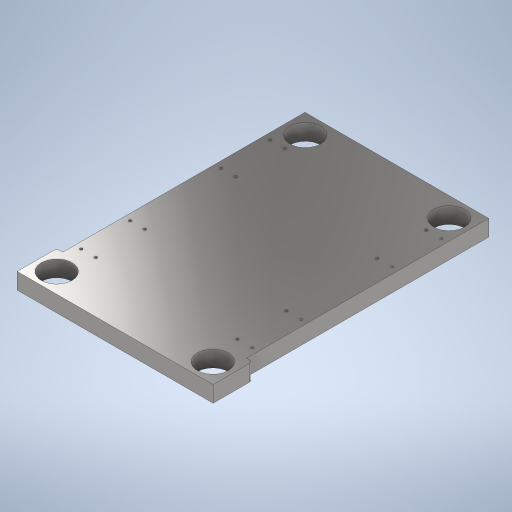
# Autodesk Inventor part: Weight Frame Top
Saved by Autodesk Inventor 2023 (Build 270158000, 158)
## iProperties
Created: 2022-10-18
Part Number: Weight Frame Top
Material: Stainless Steel
Document SubType Name: Modeling
Designer: Hayden Swanson
Density: 8 g/cm^3
Appearance: Semi-Polished
Author: Hayden Swanson
Autodesk Inventor part; units mm, degrees
ref_plane "YZ Plane" through (0, 0, 0) normal (1, 0, 0) x (0, 1, 0)
ref_plane "XZ Plane" through (0, 0, 0) normal (0, 1, 0) x (-1, 0, 0)
ref_plane "XY Plane" through (0, 0, 0) normal (0, 0, 1) x (1, 0, 0)
sketch "Sketch1" plane through (0, 0, 0) normal (0, 1, 0) x (-1, 0, 0)
  line L0 (0, 0) -> (190.5, 0)
  line L1 (190.5, 0) -> (190.5, -292.1)
  line L2 (190.5, -292.1) -> (0, -292.1)
  line L3 (0, -292.1) -> (0, 0)
  line L4 (0, -292.1) -> (-6.35, -292.1)
  line L5 (-6.35, -292.1) -> (-6.35, 0)
  line L6 (-6.35, 0) -> (0, 0)
  line L7 (190.5, -292.1) -> (196.85, -292.1)
  line L8 (196.85, -292.1) -> (196.85, 0)
  line L9 (196.85, 0) -> (190.5, 0)
  dimension "d0" = 190.5
  dimension "d1" = 292.1
  dimension "d259" = 6.35
  dimension "d260" = 6.35
  constraints: 20 end point, 4 perpendicular, 3 horizontal, 3 parallel
  measures "d0" distance of L1.end L2.end
  measures "d1" distance of L0.end L1.end
  measures "d259" distance of L2.end L4.end
  measures "d260" distance of L1.end L7.end
extrude "Extrusion1" add sketch "Sketch1" along normal blind 16.764
sketch "Sketch2" plane through (0, 16.764, 0) normal (0, 1, 0) x (1, 0, 0)
  line L0 (-176.2125, 0) -> (-176.2125, 20.32)
  line L1 (0, 0) -> (-14.2875, 0)
  line L2 (-14.2875, 0) -> (-14.2875, 20.32)
  line L3 (-190.5, 292.1) -> (-169.8625, 292.1)
  line L4 (-169.8625, 292.1) -> (-169.8625, 271.78)
  line L5 (-190.5, 271.78) -> (-190.5, 292.1)
  line L6 (0, 292.1) -> (-20.6375, 292.1)
  line L7 (-20.6375, 292.1) -> (-20.6375, 271.78)
  line L8 (0, 271.78) -> (0, 292.1)
  circle A0 centre (-176.2125, 20.32) radius 15.9766
  circle A1 centre (-14.2875, 20.32) radius 15.9766
  circle A2 centre (-20.6375, 271.78) radius 15.9766
  circle A3 centre (-169.8625, 271.78) radius 15.9766
  line L9 (6.35, 0) -> (6.35, 292.1) projected
  line L10 (6.35, 20.32) -> (-14.2875, 20.32)
  line L11 (-196.85, 292.1) -> (-196.85, 0) projected
  line L12 (-196.85, 20.32) -> (-176.2125, 20.32)
  dimension "d5" = 20.32
  dimension "d7" = 20.32
  dimension "d9" = 20.32
  dimension "d11" = 20.32
  dimension "d12" = 31.9532
  dimension "d14" = 31.9532
  dimension "d15" = 31.9532
  dimension "d264" = 31.9532
  dimension "d274" = 20.6375
  dimension "d276" = 20.6375
  constraints: 22 end point, 4 centre point, 4 coincident, 4 horizontal, 4 perpendicular, 2 parallel, 2 point on line
  measures "d5" distance of L0.end L0.start
  measures "d7" distance of L1.end L2.end
  measures "d9" distance of L3.end L4.end
  measures "d11" distance of L7.end L6.end
  measures "d12" diameter of A0
  measures "d14" diameter of A2
  measures "d15" diameter of A3
  measures "d264" diameter of A1
  measures "d274" distance of L10.start L10.end
  measures "d276" distance of L12.start L12.end
extrude "Extrusion2" cut sketch "Sketch2" against normal through all
sketch "Sketch7" plane through (0, 16.764, 0) normal (0, 1, 0) x (1, 0, 0)
  circle A0 centre (-14.2875, 20.32) radius 15.9766 projected
  line L0 (-14.2875, 53.2511) -> (-14.2875, 78.6511)
  line L1 (-14.2875, 78.6511) -> (-14.2875, 104.0511)
  line L2 (-14.2875, 53.2511) -> (-6.6675, 53.2511)
  line L3 (-14.2875, 104.0511) -> (-6.6675, 104.0511)
  line L4 (-14.2875, 104.0511) -> (-21.9075, 104.0511)
  line L5 (-14.2875, 53.2511) -> (-21.9075, 53.2511)
  line L6 (-14.2875, 198.2978) -> (-21.9075, 198.2978)
  line L7 (-14.2875, 249.0978) -> (-21.9075, 249.0978)
  line L8 (-14.2875, 198.2978) -> (-6.6675, 198.2978)
  line L9 (-14.2875, 249.0978) -> (-6.6675, 249.0978)
  circle A1 centre (-176.2125, 20.32) radius 15.9766 projected
  line L10 (-176.2125, 53.2511) -> (-176.2125, 78.6511)
  line L11 (-176.2125, 78.6511) -> (-176.2125, 104.0511)
  line L12 (-176.2125, 104.0511) -> (-176.2125, 198.2978)
  line L13 (-176.2125, 198.2978) -> (-176.2125, 223.6978)
  line L14 (-176.2125, 223.6978) -> (-176.2125, 249.0978)
  line L15 (-176.2125, 249.0978) -> (-168.5925, 249.0978)
  line L16 (-176.2125, 249.0978) -> (-183.8325, 249.0978)
  line L17 (-176.2125, 198.2978) -> (-183.8325, 198.2978)
  line L18 (-176.2125, 198.2978) -> (-168.5925, 198.2978)
  line L19 (-176.2125, 53.2511) -> (-183.8325, 53.2511)
  line L20 (-176.2125, 53.2511) -> (-168.5925, 53.2511)
  line L21 (-176.2125, 104.0511) -> (-183.8325, 104.0511)
  line L22 (-176.2125, 104.0511) -> (-168.5925, 104.0511)
  circle A2 centre (-183.8325, 53.2511) radius 1.75
  circle A3 centre (-183.8325, 104.0511) radius 1.75
  circle A4 centre (-168.5925, 53.2511) radius 1.75
  circle A5 centre (-168.5925, 104.0511) radius 1.75
  circle A6 centre (-183.8325, 198.2978) radius 1.75
  circle A7 centre (-168.5925, 198.2978) radius 1.75
  circle A8 centre (-183.8325, 249.0978) radius 1.75
  circle A9 centre (-168.5925, 249.0978) radius 1.75
  circle A10 centre (-21.9075, 53.2511) radius 1.75
  circle A11 centre (-6.6675, 53.2511) radius 1.75
  circle A12 centre (-21.9075, 104.0511) radius 1.75
  circle A13 centre (-6.6675, 104.0511) radius 1.75
  circle A14 centre (-21.9075, 198.2978) radius 1.75
  circle A15 centre (-21.9075, 249.0978) radius 1.75
  circle A16 centre (-6.6675, 198.2978) radius 1.75
  circle A17 centre (-6.6675, 249.0978) radius 1.75
  line L23 (-176.2125, 151.1745) -> (-14.2875, 151.1745)
  line L24 (-14.2875, 249.0978) -> (-14.2875, 53.2511)
  point P0 (0, 0)
  point P1 (6.35, 31.7989)
  point P2 (6.35, 8.8411)
  point P3 (-196.85, 8.8411)
  point P4 (-196.85, 31.7989)
  dimension "d167" = 25.4
  dimension "d168" = 25.4
  dimension "d169" = 94.2467
  dimension "d172" = 7.62
  dimension "d173" = 7.62
  dimension "d174" = 7.62
  dimension "d175" = 7.62
  dimension "d176" = 7.62
  dimension "d177" = 7.62
  dimension "d178" = 7.62
  dimension "d179" = 7.62
  dimension "d182" = 25.4
  dimension "d183" = 25.4
  dimension "d184" = 94.2467
  dimension "d185" = 25.4
  dimension "d186" = 25.4
  dimension "d187" = 7.62
  dimension "d188" = 7.62
  dimension "d189" = 7.62
  dimension "d190" = 7.62
  dimension "d191" = 7.62
  dimension "d192" = 7.62
  dimension "d193" = 7.62
  dimension "d194" = 7.62
  dimension "d195" = 3.5
  dimension "d196" = 3.5
  dimension "d197" = 3.5
  dimension "d198" = 3.5
  dimension "d199" = 3.5
  dimension "d200" = 3.5
  dimension "d201" = 3.5
  dimension "d202" = 3.5
  dimension "d203" = 3.5
  dimension "d204" = 3.5
  dimension "d205" = 3.5
  dimension "d206" = 3.5
  dimension "d207" = 3.5
  dimension "d208" = 3.5
  dimension "d209" = 3.5
  dimension "d210" = 3.5
  dimension "d258" = 161.925
  constraints: 50 end point, 16 centre point, 16 coincident, 14 horizontal, 4 point on line, 2 perpendicular, 1 midpoint, 2 other
  measures "d167" distance of L0.start L0.end
  measures "d168" distance of L0.end L1.end
  measures "d169" distance of L1.end L6.start
  measures "d172" distance of L0.start L2.end
  measures "d173" distance of L1.end L3.end
  measures "d174" distance of L1.end L4.end
  measures "d175" distance of L0.start L5.end
  measures "d176" distance of L6.start L6.end
  measures "d177" distance of L7.start L7.end
  measures "d178" distance of L6.start L8.end
  measures "d179" distance of L7.start L9.end
  measures "d182" distance of L10.start L10.end
  measures "d183" distance of L10.end L11.end
  measures "d184" distance of L11.end L12.end
  measures "d185" distance of L12.end L13.end
  measures "d186" distance of L13.end L14.end
  measures "d187" distance of L14.end L15.end
  measures "d188" distance of L14.end L16.end
  measures "d189" distance of L12.end L17.end
  measures "d190" distance of L12.end L18.end
  measures "d191" distance of L10.start L19.end
  measures "d192" distance of L10.start L20.end
  measures "d193" distance of L11.end L21.end
  measures "d194" distance of L11.end L22.end
  measures "d195" diameter of A2
  measures "d196" diameter of A3
  measures "d197" diameter of A4
  measures "d198" diameter of A5
  measures "d199" diameter of A6
  measures "d200" diameter of A7
  measures "d201" diameter of A8
  measures "d202" diameter of A9
  measures "d203" diameter of A10
  measures "d204" diameter of A11
  measures "d205" diameter of A12
  measures "d206" diameter of A13
  measures "d207" diameter of A14
  measures "d208" diameter of A15
  measures "d209" diameter of A16
  measures "d210" diameter of A17
  measures "d258" distance of L23.start L23.end
hole "Hole1" at (-183.8325, 16.764, -53.2511) at (-168.5925, 16.764, -53.2511) at (-183.8325, 16.764, -104.0511) at (-168.5925, 16.764, -104.0511) at (-183.8325, 16.764, -198.2978) at (-168.5925, 16.764, -198.2978) at (-183.8325, 16.764, -249.0978) at (-168.5925, 16.764, -249.0978) at (-6.6675, 16.764, -249.0978) at (-21.9075, 16.764, -249.0978) at (-6.6675, 16.764, -198.2978) at (-21.9075, 16.764, -198.2978) at (-6.6675, 16.764, -104.0511) at (-21.9075, 16.764, -104.0511) at (-6.6675, 16.764, -53.2511) at (-21.9075, 16.764, -53.2511) direction (0, -1, 0) diameter 2.85 end through all thread size "M3.5x0.6" class "6H" standard "ANSI Metric M Profile"
sketch "Sketch11" plane through (0, 16.764, 0) normal (0, 1, 0) x (1, 0, 0)
  circle A0 centre (-14.2875, 20.32) radius 15.9766 projected
  line L0 (-14.2875, 20.32) -> (-14.2875, 40.9575)
  line L1 (6.35, 292.1) -> (-196.85, 292.1) projected
  line L2 (6.35, 292.1) -> (0, 292.1)
  line L3 (0, 292.1) -> (0, 40.9575)
  line L4 (0, 40.9575) -> (6.35, 40.9575)
  line L5 (6.35, 40.9575) -> (6.35, 292.1)
  circle A1 centre (-176.2125, 20.32) radius 15.9766 projected
  line L6 (-176.2125, 20.32) -> (-176.2125, 40.9575)
  line L7 (-196.85, 292.1) -> (-196.85, 0) projected
  line L8 (-196.85, 292.1) -> (-190.5, 292.1)
  line L9 (-190.5, 292.1) -> (-190.5, 40.9575)
  line L10 (-190.5, 40.9575) -> (-196.85, 40.9575)
  line L11 (-196.85, 40.9575) -> (-196.85, 292.1)
  point P0 (0, 0)
  point P1 (-196.85, 40.9575)
  point P2 (6.35, 31.7989)
  point P3 (6.35, 8.8411)
  point P4 (-196.85, 8.8411)
  point P5 (-196.85, 31.7989)
  dimension "d266" = 20.6375
  dimension "d267" = 20.6375
  dimension "d272" = 6.35
  dimension "d273" = 6.35
  constraints: 20 end point, 4 parallel, 2 horizontal, 2 perpendicular, 2 vertical, 2 other
  measures "d266" distance of L0.start L0.end
  measures "d267" distance of L6.start L6.end
  measures "d272" distance of L3.end L4.end
  measures "d273" distance of L9.end L10.end
extrude "Extrusion10" cut sketch "Sketch11" against normal blind 16.764 contours L5 L4 L3 L1 | L9 L10 L7 L1
fillet "Fillet5" radius 3.175 2 edges at (-196.85, 8.382, -40.9575) (6.35, 8.382, -40.9575)
body "Solid1"
